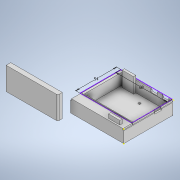
# Autodesk Inventor part: Shell 2 top
Saved by Autodesk Inventor 2022 (Build 260153000, 153)
## iProperties
Created: 2021-10-12
Part Number: Shell 2 top
Material: Generic
Document SubType Name: Modeling
Designer: Elisabeth
Density: 1 g/cm^3
Appearance: Default
Author: Elisabeth
Autodesk Inventor part; units mm, degrees
ref_plane "YZ Plane" through (0, 0, 0) normal (1, 0, 0) x (0, 1, 0)
ref_plane "XZ Plane" through (0, 0, 0) normal (0, 1, 0) x (-1, 0, 0)
ref_plane "XY Plane" through (0, 0, 0) normal (0, 0, 1) x (1, 0, 0)
sketch "Sketch1" plane through (0, 0, 0) normal (0, 1, 0) x (-1, 0, 0)
  point P0 (0, 0)
sketch "Sketch2" plane through (0, 0, 0) normal (0, 1, 0) x (-1, 0, 0)
  line L0 (70, 0) -> (70, -66)
  line L1 (70, -66) -> (0, -66)
  line L2 (0, -66) -> (0, 0)
  line L3 (70, 0) -> (0, 0)
  point P0 (0, 0)
  dimension "d0" = 70
  dimension "d138" = 66
  constraints: 8 end point, 1 parallel, 1 perpendicular
  measures "d0" distance of L0.end L1.end
  measures "d138" distance between parallel lines of L3 L1
extrude "Extrusion1" add sketch "Sketch2" along normal blind 16.75
sketch "Sketch3" plane through (0, 16.75, 0) normal (0, 1, 0) x (1, 0, 0)
  line L0 (0, 66) -> (-70, 66) projected
  line L1 (-70, 66) -> (-2, 66)
  line L2 (-70, 66) -> (-2, 66)
  line L3 (-2, 66) -> (-70, 66)
  line L4 (-70, 66) -> (-70, 12)
  line L5 (-70, 12) -> (-2, 12)
  line L6 (-2, 66) -> (-2, 12)
  point P0 (0, 0)
  dimension "d135" = 68
  dimension "d136" = 54
  constraints: 12 end point, 3 perpendicular, 1 point on line
  measures "d135" distance of L2.end L3.end
  measures "d136" distance of L3.end L4.end
sketch "Sketch4" plane through (0, 16.75, 0) normal (0, 1, 0) x (1, 0, 0)
  line L0 (0, 66) -> (-70, 66) projected
  line L1 (-30.4814, 66) -> (-28.4814, 66)
  line L2 (-28.4814, 66) -> (-28.4814, 64)
  line L3 (-70, 66) -> (-70, 0) projected
  line L4 (-70, 37.8423) -> (-70, 39.8423)
  line L5 (-70, 39.8423) -> (-68, 39.8423)
  line L6 (0, 38.8423) -> (0, 36.8423)
  line L7 (0, 36.8423) -> (-2, 36.8423)
  line L8 (-66, 64) -> (-2, 64)
  line L9 (-2, 64) -> (-2, 14)
  line L10 (-2, 14) -> (-66, 14)
  line L11 (-66, 14) -> (-66, 64)
  dimension "d5" = 2
  dimension "d6" = 2
  dimension "d7" = 2
  dimension "d11" = 2
  dimension "d75" = 2
  dimension "d132" = 50
  dimension "d133" = 64
  constraints: 20 end point, 4 perpendicular, 4 point on line, 2 parallel, 1 horizontal
  measures "d5" distance of L1.start L1.end
  measures "d6" distance of L1.end L2.end
  measures "d7" distance of L4.start L4.end
  measures "d11" distance of L6.start L6.end
  measures "d75" distance between parallel lines of L0 L8
  measures "d132" distance between parallel lines of L8 L10
  measures "d133" distance of L8.start L8.end
extrude "Extrusion2" cut sketch "Sketch4" against normal blind 14.75
sketch "Sketch7" plane through (0, 16.75, 0) normal (0, 1, 0) x (1, 0, 0)
  line L0 (-70, 66) -> (-69, 66)
  line L1 (-70, 66) -> (-6, 66)
  line L2 (-70, 65) -> (-70, 66)
  line L3 (0, 66) -> (-7, 66)
  line L4 (-69, 65) -> (-1, 65)
  line L5 (0, 66) -> (-70, 66) projected
  line L6 (-70, 66) -> (0, 66)
  line L7 (0, 0) -> (0, 66) projected
  line L8 (0, 0) -> (-1, 0)
  line L9 (-1, 66) -> (0, 66)
  line L10 (0, 66) -> (0, 0)
  line L11 (0, 0) -> (-1, 0)
  line L12 (-70, 0) -> (0, 0) projected
  line L13 (-1, 65) -> (-1, 0)
  line L14 (0, 0) -> (-1, 0)
  line L15 (-69, 65) -> (-69, 0)
  line L16 (-70, 66) -> (-70, 0) projected
  line L17 (-69, 0) -> (-70, 0)
  line L18 (-70, 0) -> (-70, 66)
  dimension "d76" = 1
  dimension "d139" = 1
  dimension "d140" = 1
  constraints: 30 end point, 6 horizontal, 3 collinear, 2 parallel, 2 perpendicular, 2 point on line
  measures "d76" distance between parallel lines of L1 L4
  measures "d139" distance between parallel lines of L7 L13
  measures "d140" distance between parallel lines of L16 L15
extrude "Extrusion3" cut sketch "Sketch7" against normal blind 2 contours L0 L1 L3 L7 L8 L13 L4 L15 L12 L16 L2
sketch "Sketch8" plane through (0, 16.75, 0) normal (0, 1, 0) x (1, 0, 0)
  line L0 (0, 12) -> (0, 13)
  line L1 (0, 13) -> (-68, 13)
  line L2 (0, 12) -> (-68, 12)
  line L3 (-68, 12) -> (-68, 13)
  line L4 (-69, 0) -> (-1, 0) projected
  point P0 (0, 0)
  point P1 (-70, 0)
  dimension "d46" = 68
  dimension "d141" = 1
  constraints: 8 end point, 1 horizontal, 1 perpendicular
  measures "d46" distance of L1.end L0.end
  measures "d141" distance of L0.start L0.end
extrude "Extrusion4" cut sketch "Sketch8" against normal blind 2
sketch "Sketch10" plane through (0, 2, 0) normal (0, 1, 0) x (1, 0, 0)
  line L0 (-31, 2) -> (-41, 2)
  line L1 (-63, 64) -> (-48, 64)
  line L2 (-48, 64) -> (-48, 61)
  line L3 (-48, 61) -> (-63, 61)
  line L4 (-63, 61) -> (-63, 64)
  line L5 (-22, 2) -> (-7, 2)
  line L6 (-7, 2) -> (-7, 5)
  line L7 (-7, 5) -> (-22, 5)
  line L8 (-22, 5) -> (-22, 2)
  line L9 (-66, 14) -> (-66, 64) projected
  line L10 (-2, 14) -> (-66, 14) projected
  line L11 (-66, 64) -> (-2, 64)
  line L12 (-2, 64) -> (-2, 14)
  line L13 (-2, 14) -> (-66, 14)
  line L14 (-66, 14) -> (-66, 64)
  point P0 (0, 0)
  point P1 (-21, 64)
  dimension "d57" = 15
  dimension "d58" = 3
  dimension "d61" = 15
  dimension "d79" = 3
  constraints: 26 end point, 6 parallel, 4 horizontal, 3 perpendicular, 1 other
  measures "d57" distance of L2.end L3.end
  measures "d58" distance of L1.end L2.end
  measures "d61" distance of L7.end L6.end
  measures "d79" distance between parallel lines of L7 L5
extrude "Extrusion5" add sketch "Sketch10" along normal blind 20 contours L1 L2 L3 L4 | L8 L7 L6 L5
sketch "Sketch11" plane through (0, 0, 0) normal (0, -1, 0) x (1, 0, 0)
  circle A0 centre (-12, -42.73) radius 3.5
  circle A1 centre (-33.5, -54.23) radius 1.5
  line L0 (0, 0) -> (0, -66) projected
  line L1 (0, -66) -> (-70, -66) projected
  line L2 (-2, -64) -> (-2, -14) projected
  dimension "d85" = 23.27
  dimension "d86" = 21.5
  dimension "d88" = 7
  dimension "d89" = 3
  dimension "d119" = 11.5
  dimension "d120" = 10
  constraints: 2 centre point
  measures "d85" distance from line of L1 A0.centre
  measures "d86" horizontal distance of A1.centre A0.centre
  measures "d88" diameter of A0
  measures "d89" diameter of A1
  measures "d119" vertical distance of A1.centre A0.centre
  measures "d120" distance from line of L2 A0.centre
extrude "Extrusion6" cut sketch "Sketch11" against normal blind 9
sketch "Sketch12" plane through (0, 0, 0) normal (0, -1, 0) x (1, 0, 0)
  line L0 (-70, 0) -> (-70, -66) projected
  line L1 (-69, 12) -> (-69, 18)
  line L2 (-69, 18) -> (-137, 18)
  line L3 (-137, 18) -> (-137, 12)
  line L4 (-137, 12) -> (-69, 12)
  line L5 (0, 0) -> (-70, 0) projected
  line L6 (0, 0) -> (-137.0429, 0)
  point P0 (-70, 0)
  dimension "d81" = 6
  dimension "d143" = 68
  dimension "d144" = 12
  constraints: 10 end point, 2 perpendicular, 1 horizontal, 1 parallel
  measures "d81" distance of L1.end L1.start
  measures "d143" distance of L1.end L2.end
  measures "d144" distance between parallel lines of L5 L4
extrude "Extrusion7" add sketch "Sketch12" against normal blind 30
sketch "Sketch13" plane through (-70, 0, 6) normal (0, 0, 1) x (1, 0, 0)
  line L0 (0, 0) -> (0, 30) projected
  line L1 (70, 0) -> (70, 14.75) projected
  line L2 (0, 30) -> (70, 30) projected
  line L3 (35, 30) -> (35, 0)
  line L4 (0, 15) -> (70, 15)
  circle A0 centre (35, 15) radius 3.175
  point P0 (0, 14.75)
  point P1 (70, 16.75)
  dimension "d91" = 6.35
  constraints: 4 end point, 3 midpoint, 1 centre point, 1 horizontal, 1 vertical
  measures "d91" diameter of A0
hole "Hole1" [suppressed]
sketch "Sketch14" plane through (0, 0, -66) normal (0, 0, -1) x (-1, 0, 0)
  line L0 (5, 16.95) -> (13.5, 16.95)
  line L1 (13.5, 16.95) -> (13.5, 12.95)
  line L2 (13.5, 12.95) -> (5, 12.95)
  line L3 (5, 12.95) -> (5, 16.95)
  line L4 (20.1, 16.95) -> (28.6, 16.95)
  line L5 (28.6, 16.95) -> (28.6, 12.95)
  line L6 (28.6, 12.95) -> (20.1, 12.95)
  line L7 (20.1, 12.95) -> (20.1, 16.95)
  line L8 (70, 14.75) -> (0, 14.75) projected
  line L9 (0, 0) -> (0, 14.75) projected
  point P0 (0, 16.75)
  dimension "d99" = 8.5
  dimension "d100" = 8.5
  dimension "d101" = 4
  dimension "d103" = 13.5
  dimension "d104" = 28.6
  dimension "d105" = 1.8
  constraints: 16 end point, 4 parallel, 2 horizontal, 2 perpendicular, 2 point on line
  measures "d99" distance of L1.end L2.end
  measures "d100" distance of L5.end L6.end
  measures "d101" distance of L2.end L0.start
  measures "d103" distance between parallel lines of L9 L1
  measures "d104" distance between parallel lines of L9 L5
  measures "d105" distance between parallel lines of L6 L8
extrude "Extrusion8" cut sketch "Sketch14" against normal blind 10
sketch "Sketch15" plane through (0, 0, -66) normal (1, 0, 0) x (0, 0, -1)
  line L0 (-25, 18.25) -> (-16, 18.25)
  line L1 (-16, 18.25) -> (-16, 13.25)
  line L2 (-16, 13.25) -> (-25, 13.25)
  line L3 (-25, 13.25) -> (-25, 18.25)
  line L4 (-78, 0) -> (-78, 30) projected
  line L5 (0, 0) -> (0, 14.75) projected
  line L6 (0, 0) -> (-84, 0) projected
  line L7 (0, 14.75) -> (-66, 14.75) projected
  point P0 (-66, 0)
  point P1 (0, 16.75)
  dimension "d108" = 9
  dimension "d109" = 5
  dimension "d111" = 25
  dimension "d113" = 1.5
  constraints: 8 end point, 2 parallel, 1 horizontal, 1 perpendicular, 1 other
  measures "d108" distance of L1.end L2.end
  measures "d109" distance of L0.end L1.end
  measures "d111" distance between parallel lines of L5 L3
  measures "d113" distance between parallel lines of L7 L2
extrude "Extrusion9" cut sketch "Sketch15" against normal blind 10
thread "Thread1" size "M7x1" class "6H" standard "ANSI Metric M Profile" full length
fillet "Fillet7" radius 2 1 edges at (0, 7.375, -66)
fillet "Fillet8" radius 2 1 edges at (-70, 7.375, -66)
fillet "Fillet9" radius 2 1 edges at (-69, 15, 18)
fillet "Fillet10" [suppressed]
body "Solid1"
